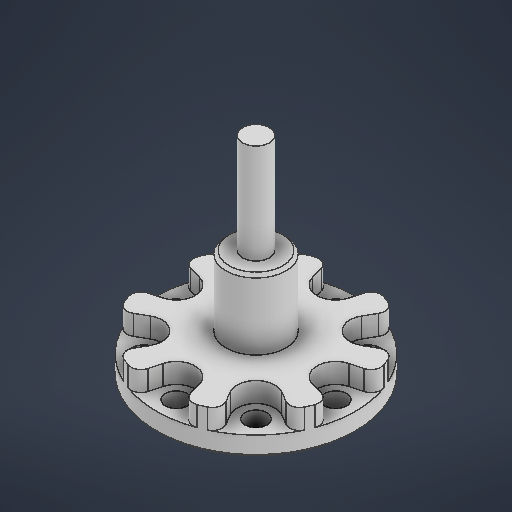
# Autodesk Inventor part: Ось шарнира
Saved by Autodesk Inventor 2025 (Build 290162010, 162A)
## iProperties
Created: 2025-01-17
Part Number: Ось шарнира
Material: Типовые
Document SubType Name: Modeling
Designer: Edward_Higgins
Density: 1 g/cm^3
Appearance: По умолчанию
Author: Edward_Higgins
Autodesk Inventor part; units mm, degrees
ref_plane "YZ Plane" through (0, 0, 0) normal (1, 0, 0) x (0, 1, 0)
ref_plane "XZ Plane" through (0, 0, 0) normal (0, 1, 0) x (-1, 0, 0)
ref_plane "XY Plane" through (0, 0, 0) normal (0, 0, 1) x (1, 0, 0)
sketch "Эскиз1" plane through (0, 0, 0) normal (0, 0, 1) x (1, 0, 0)
  line L0 (0, 11) -> (3, 11)
  line L1 (3, 11) -> (3, 2)
  line L2 (3, 2) -> (10, 2)
  line L3 (10, 2) -> (10, 0)
  line L4 (10, 0) -> (0, 0)
  line L5 (0, 0) -> (0, 11)
  dimension "d0" = 6
  dimension "d1" = 2
  dimension "d2" = 20
  dimension "d3" = 9
  constraints: 12 end point, 5 perpendicular, 1 horizontal
  measures "d0" diameter of L1 L5
  measures "d1" distance of L2.end L3.end
  measures "d2" diameter of L3 L5
  measures "d3" distance of L0.end L1.end
revolve "Вращение1" add sketch "Эскиз1" angle 360 about axis through (0, 0, 0) along (0, 1, 0)
sketch "Эскиз2" plane through (0, 2, 0) normal (0, 1, 0) x (1, 0, 0)
  circle A0 centre (8, 0) radius 1.1
  point P0 (0, 0)
  dimension "d5" = 2.2
  dimension "d6" = 8
  constraints: 1 centre point, 1 horizontal alignment
  measures "d5" diameter of A0
  measures "d6" distance of A0.centre point (0, 0)
extrude "Выдавливание1" cut sketch "Эскиз2" against normal up to surface (2 mm away)
pattern_circular "Круговой массив1" count 8 over 360 about axis through (0, 1, 0) along (0, 1, 0) of "Выдавливание1"
chamfer "Фаска1" distance 0.3 angle 45 2 edges at (-3, 11, 0) (-10, 0, 0)
sketch "Эскиз3" plane through (0, 2, 0) normal (0, 1, 0) x (1, 0, 0)
  circle A0 centre (-8, 0) radius 1.1 projected
  arc A1 (-7.5121, -1.8208) -> (-7.5121, 1.8208) centre (-8, 0) ccw
  line L0 (-7.5121, 1.8208) -> (-9.7056, 2.4085)
  line L1 (-7.5121, -1.8208) -> (-9.7056, -2.4085)
  circle A2 centre (0, 0) radius 10 projected
  circle A3 centre (5.6569, -5.6569) radius 1.1 projected
  circle A4 centre (0, -8) radius 1.1 projected
  circle A5 centre (-5.6569, -5.6569) radius 1.1 projected
  circle A6 centre (-8, 0) radius 1.1 projected
  circle A7 centre (-5.6569, 5.6569) radius 1.1 projected
  circle A8 centre (0, 8) radius 1.1 projected
  circle A9 centre (5.6569, 5.6569) radius 1.1 projected
  circle A10 centre (8, 0) radius 1.1 projected
  circle A11 centre (0, 0) radius 3 projected
  circle A12 centre (0, 0) radius 10 projected
  dimension "d15" = 3.77
  dimension "d24" = 30
  constraints: 4 end point, 4 point on circle, 2 tangent, 1 centre point, 1 coincident, 1 vertical alignment, 2 other
  measures "d15" diameter of A1
  measures "d24" angle of L1 L0
extrude "Выдавливание2" add sketch "Эскиз3" along normal blind 2
extrude "Выдавливание3" cut sketch "Эскиз3" along normal up to surface (2 mm away) contours L1 A2 L0 A1 picked at (-8.5359, -1.7526)
fillet "Сопряжение1" radius 1 2 edges at (-9.7056, 3, -2.4085) (-9.7056, 3, 2.4085)
pattern_circular "Круговой массив2" count 8 over 360 about axis through (0, 6.5, 0) along (0, 1, 0) of "Выдавливание3", "Сопряжение1"
sketch "Эскиз4" plane through (0, 11, 0) normal (0, 1, 0) x (1, 0, 0)
  circle A0 centre (0, 0) radius 1.3421
  constraints: 1 centre point, 1 coincident
extrude "Выдавливание4" add sketch "Эскиз4" along normal blind 10
